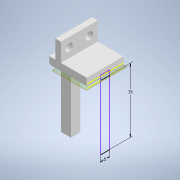
# Autodesk Inventor part: reverse_finger
Saved by Autodesk Inventor 2021 (Build 250183000, 183)
## iProperties
Created: 2023-04-10
Part Number: reverse_finger
Material: Generic
Document SubType Name: Modeling
Designer: mahmo
Density: 1 g/cm^3
Appearance: Default
Author: mahmo
Autodesk Inventor part; units mm, degrees
ref_plane "YZ Plane" through (0, 0, 0) normal (1, 0, 0) x (0, 1, 0)
ref_plane "XZ Plane" through (0, 0, 0) normal (0, 1, 0) x (-1, 0, 0)
ref_plane "XY Plane" through (0, 0, 0) normal (0, 0, 1) x (1, 0, 0)
sketch "Sketch1" plane through (0, 0, 0) normal (1, 0, 0) x (0, 1, 0)
  line L0 (-2.5, 10) -> (2.5, 10)
  line L1 (2.5, 10) -> (2.5, -10)
  line L2 (2.5, -10) -> (-2.5, -10)
  line L3 (-2.5, -10) -> (-2.5, 10)
  line L4 (-2.5, 10) -> (2.5, -10) construction
  line L5 (2.5, 10) -> (-2.5, -10) construction
  point P0 (0, 0)
  dimension "d0" = 5
  dimension "d1" = 20
  constraints: 12 end point, 2 midpoint, 2 parallel, 1 horizontal, 1 perpendicular
  measures "d0" distance of L1.end L2.end
  measures "d1" distance of L0.end L1.end
extrude "Extrusion1" add sketch "Sketch1" along normal blind 17
sketch "Sketch3" plane through (0, -2.5, 10) normal (0, 0, 1) x (1, 0, 0)
  line L0 (3, 5) -> (0, 5)
  line L1 (0, 5) -> (0, 15)
  line L2 (0, 15) -> (3, 15)
  line L3 (3, 15) -> (3, 5)
  point P0 (0, 2.5)
  dimension "d8" = 3
  dimension "d9" = 10
  constraints: 8 end point, 2 parallel, 1 horizontal, 1 perpendicular, 1 other
  measures "d8" distance of L1.end L2.end
  measures "d9" distance of L0.end L1.end
extrude "Extrusion3" add sketch "Sketch3" against normal up to surface (20 mm away)
sketch "Sketch4" plane through (0, 0, 0) normal (-1, 0, 0) x (0, 0, 1)
  circle A0 centre (-121.4441, 7.5) radius 2 projected
  circle A1 centre (-132.4441, 7.5) radius 2 projected
  point P0 (0, 0)
extrude "Extrusion4" cut sketch "Sketch4" against normal through all
sketch "Sketch5" plane through (0, 0, 0) normal (-1, 0, 0) x (0, 0, 1)
  line L0 (-2.5, -37.5) -> (-2.5, -2.5) projected
  line L1 (-10, -2.5) -> (10, -2.5) projected
  line L2 (2.5, -2.5) -> (2.5, -37.5) projected
  line L3 (2.5, -37.5) -> (-2.5, -37.5) projected
  point P0 (0, 0)
extrude "Extrusion5" add sketch "Sketch5" against normal blind 5
sketch "Sketch6" plane through (0, 0, 0) normal (-1, 0, 0) x (0, 0, 1)
  circle A0 centre (-5.5, 7.5) radius 2 projected
  circle A1 centre (5.5, 7.5) radius 2 projected
  point P0 (0, 0)
extrude "Extrusion6" cut sketch "Sketch6" against normal blind 10
ref_plane "Work Plane1" through (0, -2.5, -10) normal (0, -1, 0) x (1, 0, 0)
split_face "Split1"
sketch "Sketch7" plane through (0, -2.5, 2.5) normal (-1, 0, 0) x (0, 0, 1)
  line L0 (-12.5, 5) -> (7.5, 5) projected
  line L1 (-5, 0) -> (0, 0) projected
  line L2 (7.5, 0) -> (0, 0) projected
  line L3 (7.5, 15) -> (7.5, 0) projected
  line L4 (7.5, 15) -> (-12.5, 15) projected
  line L5 (-12.5, 0) -> (-12.5, 15) projected
  line L6 (-5, 0) -> (-12.5, 0) projected
  circle A0 centre (3, 10) radius 2 projected
  circle A1 centre (-8, 10) radius 2 projected
  line L7 (-5, 0) -> (0, 0) projected
  line L8 (-5, 0) -> (-5, -35) projected
  line L9 (-5, -35) -> (0, -35) projected
  line L10 (0, -35) -> (0, 0) projected
  point P0 (-2.5, 2.5)
extrude "Extrusion7" add sketch "Sketch7" along normal blind 4 contours L0 L3 L2 L1 L6 L5 | L1 L10 L9 L8
sketch "Sketch8" plane through (5, 0, 0) normal (1, 0, 0) x (0, 0, -1)
  line L0 (-2.5, -2.5) -> (-2.5, -37.5) projected
  line L1 (-2.5, -37.5) -> (2.5, -37.5) projected
  line L2 (2.5, -37.5) -> (2.5, -2.5) projected
  line L3 (-2.5, -2.5) -> (2.5, -2.5) projected
  point P0 (0, 0)
extrude "Extrusion8" cut sketch "Sketch8" against normal blind 4
move faces "Move1" translate (-0.5, 0, 0) faces at (-4, -14.1667, 0.8333)
fillet "Fillet3" radius 2 6 edges at (6.25, -2.5, -10) (17, -2.5, 0) (6.25, -2.5, 10) (-4.5, 0, 10) (-4.5, 2.5, 0) (-4.5, 0, -10)
fillet "Fillet4" radius 2 4 edges at (-4.5, -2.5, 5.25) (-3.9142, -1.9142, 9.4142) (-4.5, -2.5, -5.25) (-3.9142, -1.9142, -9.4142)
sketch "Sketch11" plane through (15, -2.5, -8) normal (0, -1, 0) x (1, 0, 0)
  point P0 (-15, 8)
sketch "Sketch2" plane through (17, 0, 0) normal (1, 0, 0) x (0, 0, -1)
  line L0 (-2.4746, -2.5) -> (2.5254, -2.5)
  line L1 (2.5254, -2.5) -> (2.5254, -37.5)
  line L2 (2.5254, -37.5) -> (-2.4746, -37.5)
  line L3 (-2.4746, -37.5) -> (-2.4746, -2.5)
  line L4 (-10, -2.5) -> (10, -2.5) projected
  line L5 (2.5254, -2.5) -> (2.5254, 0)
  line L6 (-2.4746, -2.5) -> (-2.4746, -0.5)
  line L7 (10, -0.5) -> (-10, -0.5) projected
  line L8 (2.5254, 0) -> (-2.2155, 0)
  line L9 (-2.4746, -0.5) -> (-2.4746, 0)
  line L10 (-2.4746, 0) -> (-2.1408, 0)
  point P0 (0, 0)
  dimension "d4" = 5
  dimension "d5" = 35
  constraints: 18 end point, 3 perpendicular, 3 point on line, 2 parallel, 2 vertical, 1 horizontal
  measures "d4" distance of L1.end L2.end
  measures "d5" distance of L0.end L1.end
sketch "Sketch12" plane through (15, -2.5, -8) normal (0, -1, 0) x (1, 0, 0)
  point P0 (-15, 8)
body "Solid1"
